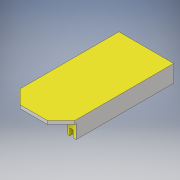
# Autodesk Inventor part: top-slider
Saved by Autodesk Inventor 2018 (Build 220112000, 112)
## iProperties
Created: 2019-10-14
Part Number: top-slider
Material: Generic
Document SubType Name: Modeling
Designer: jklei
Density: 1 g/cm^3
Appearance: Default
Author: jklei
Autodesk Inventor part; units mm, degrees
ref_plane "YZ Plane" through (0, 0, 0) normal (1, 0, 0) x (0, 1, 0)
ref_plane "XZ Plane" through (0, 0, 0) normal (0, 1, 0) x (-1, 0, 0)
ref_plane "XY Plane" through (0, 0, 0) normal (0, 0, 1) x (1, 0, 0)
sketch "Sketch1" plane through (0, 0, 0) normal (0, 0, 1) x (1, 0, 0)
  line L0 (0, 0) -> (0, 6.35)
  line L1 (0, 6.35) -> (-3.048, 6.35)
  line L2 (44.831, 15.875) -> (-5.969, 15.875)
  line L3 (1.905, 0) -> (1.905, 12.7)
  line L4 (-3.048, 0) -> (-5.969, 0)
  line L5 (-5.969, 0) -> (-5.969, 15.875)
  line L6 (44.831, 0) -> (41.91, 0)
  line L7 (41.91, 6.35) -> (38.862, 6.35)
  line L8 (38.862, 6.35) -> (38.862, 0)
  line L9 (38.862, 0) -> (36.957, 0)
  line L10 (36.957, 0) -> (36.957, 12.7)
  line L11 (0, 0) -> (1.905, 0)
  line L12 (44.831, 0) -> (44.831, 15.875)
  line L13 (1.905, 12.7) -> (36.957, 12.7)
  line L14 (-3.048, 6.35) -> (-3.048, 0)
  line L15 (41.91, 6.35) -> (41.91, 0)
  dimension "d3" = 6.35
  dimension "d4" = 3.048
  dimension "d9" = 1.905
  dimension "d10" = 12.7
  dimension "d15" = 50.8
  dimension "d18" = 15.875
  dimension "d19" = 15.875
  dimension "d21" = 6.35
  dimension "d22" = 3.048
  dimension "d23" = 1.905
  dimension "d24" = 12.7
  dimension "d25" = 35.052
  dimension "d26" = 2.921
  dimension "d27" = 2.921
  constraints: 32 end point, 5 perpendicular, 4 horizontal, 4 vertical
  measures "d3" distance of L0.start L0.end
  measures "d4" distance of L0.end L1.end
  measures "d9" distance of L0.start L3.start
  measures "d10" distance of L3.start L3.end
  measures "d15" distance of L2.start L2.end
  measures "d18" distance of L2.start L6.start
  measures "d19" distance of L4.end L2.end
  measures "d21" distance of L6.end L7.start
  measures "d22" distance of L7.start L7.end
  measures "d23" distance of L8.end L9.end
  measures "d24" distance of L9.end L10.end
  measures "d25" distance of L3.end L10.end
  measures "d26" distance of L4.start L4.end
  measures "d27" distance of L6.start L6.end
extrude "Extrusion1" add sketch "Sketch1" along normal blind 91.44
sketch "Sketch2" plane through (0, 0, 91.44) normal (0, 0, 1) x (1, 0, 0)
  line L0 (44.831, 15.875) -> (-5.969, 15.875) projected
  line L1 (44.831, 0) -> (44.831, 15.875) projected
  line L2 (-5.969, 15.875) -> (44.831, 15.875)
  line L3 (44.831, 15.875) -> (44.831, 12.7)
  line L4 (44.831, 12.7) -> (-5.969, 12.7)
  line L5 (-5.969, 12.7) -> (-5.969, 15.875)
  point P0 (0, 0)
  dimension "d28" = 3.175
  constraints: 8 end point, 2 parallel, 1 horizontal, 1 perpendicular, 1 point on line
  measures "d28" distance of L2.end L3.end
extrude "Extrusion2" add sketch "Sketch2" along normal blind 14.0208
chamfer "Chamfer1" distance 12.7 angle 45 2 edges at (44.831, 14.2875, 105.4608) (-5.969, 14.2875, 105.4608)
sketch "Sketch3" plane through (0, 0, 0) normal (0, 0, -1) x (-1, 0, 0)
  line L0 (0, 0) -> (0, 6.35) projected
  line L1 (0, 6.35) -> (3.048, 6.35) projected
  line L2 (3.048, 6.35) -> (3.048, 0) projected
  line L3 (3.048, 0) -> (5.969, 0) projected
  line L4 (5.969, 0) -> (5.969, 15.875) projected
  line L5 (5.969, 15.875) -> (-44.831, 15.875) projected
  line L6 (-44.831, 15.875) -> (-44.831, 0) projected
  line L7 (-44.831, 0) -> (-41.91, 0) projected
  line L8 (-41.91, 0) -> (-41.91, 6.35) projected
  line L9 (-41.91, 6.35) -> (-38.862, 6.35) projected
  line L10 (-38.862, 6.35) -> (-38.862, 0) projected
  line L11 (-38.862, 0) -> (-36.957, 0) projected
  line L12 (-36.957, 0) -> (-36.957, 12.7) projected
  line L13 (-36.957, 12.7) -> (-1.905, 12.7) projected
  line L14 (-1.905, 12.7) -> (-1.905, 0) projected
  line L15 (-1.905, 0) -> (0, 0) projected
extrude "Extrusion3" cut sketch "Sketch3" against normal blind 3.81
sketch "Sketch4" plane through (0, 0, 3.81) normal (0, 0, -1) x (-1, 0, 0)
  line L0 (-44.831, 12.7) -> (-44.831, 15.875) projected
  line L1 (5.969, 0) -> (-44.831, 0)
  line L2 (-44.831, 0) -> (-44.831, 15.875)
  line L3 (-44.831, 15.875) -> (5.969, 15.875)
  line L4 (5.969, 15.875) -> (5.969, 0)
  point P0 (0, 0)
  constraints: 8 end point, 2 parallel, 1 horizontal, 1 perpendicular
extrude "Extrusion4" add sketch "Sketch4" along normal blind 2.54
body "Solid1"
